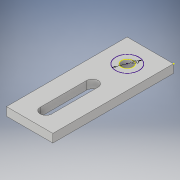
# Autodesk Inventor part: WireHangerBase
Saved by Autodesk Inventor 2018 (Build 220112000, 112)
## iProperties
Created: 2017-12-01
Part Number: WireHangerBase
Material: Generic
Document SubType Name: Modeling
Designer: ball
Density: 1 g/cm^3
Appearance: Default
Author: ball
Autodesk Inventor part; units mm, degrees
ref_plane "YZ Plane" through (0, 0, 0) normal (1, 0, 0) x (0, 1, 0)
ref_plane "XZ Plane" through (0, 0, 0) normal (0, 1, 0) x (-1, 0, 0)
ref_plane "XY Plane" through (0, 0, 0) normal (0, 0, 1) x (1, 0, 0)
sketch "Sketch1" plane through (0, 0, 0) normal (0, 1, 0) x (-1, 0, 0)
  line L0 (0, 0) -> (12.7, 0)
  line L1 (12.7, 0) -> (12.7, 33.02)
  line L2 (12.7, 33.02) -> (0, 33.02)
  line L3 (0, 33.02) -> (0, 0)
  dimension "d0" = 12.7
  dimension "d1" = 33.02
  constraints: 8 end point, 2 parallel, 1 horizontal, 1 perpendicular
  measures "d0" distance of L2.end L1.end
  measures "d1" distance of L1.end L0.end
extrude "Extrusion1" add sketch "Sketch1" along normal blind 2.286
sketch "Sketch2" plane through (0, 2.286, 0) normal (0, 1, 0) x (1, 0, 0)
  point P0 (0, 0)
sketch "Sketch3" plane through (0, 2.286, 0) normal (0, 1, 0) x (1, 0, 0)
  circle A0 centre (-6.35, -6.35) radius 1.778
  point P0 (0, 0)
  dimension "d4" = 3.556
  constraints: 1 centre point
  measures "d4" diameter of A0
hole "Hole1" at (-6.35, 2.286, 6.35) direction (0, -1, 0) diameter 3.175 end through all
sketch "Sketch4" plane through (0, 2.286, 0) normal (0, 1, 0) x (1, 0, 0)
  point P0 (0, 0)
sketch "Sketch6" plane through (0, 2.286, 0) normal (0, 1, 0) x (1, 0, 0)
  line L0 (-6.35, -15.875) -> (-6.35, -28.575) construction
  line L1 (-7.9375, -15.875) -> (-7.9375, -28.575)
  line L2 (-4.7625, -28.575) -> (-4.7625, -15.875)
  arc A0 (-4.7625, -15.875) -> (-7.9375, -15.875) centre (-6.35, -15.875) ccw
  arc A1 (-7.9375, -28.575) -> (-4.7625, -28.575) centre (-6.35, -28.575) ccw
  point P0 (0, 0)
  point P1 (-6.35, -12.7)
  point P2 (-6.35, -22.225)
  dimension "d15" = 3.175
  constraints: 8 end point, 4 point on circle, 4 tangent, 2 centre point, 1 midpoint, 1 parallel, 1 vertical
  measures "d15" diameter of A1
extrude "Extrusion3" cut sketch "Sketch6" against normal blind 2.286
sketch "Sketch7" plane through (0, 2.286, 0) normal (0, 1, 0) x (1, 0, 0)
  circle A0 centre (-6.35, -6.35) radius 1.5875 projected
  circle A1 centre (-6.35, -6.35) radius 3.175
  point P0 (0, 0)
  dimension "d18" = 6.35
  constraints: 1 centre point, 1 coincident
  measures "d18" diameter of A1
body "Solid1"
